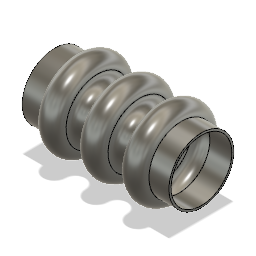
Table_13p3_Problem_6b (Autodesk Fusion 360 design; units mm, degrees)
Autodesk Fusion 360 part; units mm, degrees
sketch "Sketch1" plane through (0, 0, 0) normal (0, 0, 1) x (1, 0, 0)
  line L0 (0, 0) -> (0, 80) construction
  line L1 (0, 0) -> (10, 0) construction
  line L2 (10, 0) -> (80, 0) construction
  line L3 (140, 60) -> (100, 60) construction
  arc A0 (100, 60) -> (60, 60) centre (80, 60) ccw construction
  arc A1 (20, 60) -> (60, 60) centre (40, 60) ccw construction
  arc A2 (20, 60) -> (0, 80) centre (0, 60) ccw construction
  line L4 (140, 60) -> (0, 60) construction
  line L5 (140, 62) -> (101.9089, 62)
  arc A3 (101.9089, 62) -> (58, 60) centre (80, 60) ccw
  arc A4 (22, 60) -> (58, 60) centre (40, 60) ccw
  arc A5 (22, 60) -> (0, 82) centre (0, 60) ccw
  line L6 (140, 58) -> (97.8885, 58)
  arc A6 (97.8885, 58) -> (62, 60) centre (80, 60) ccw
  arc A7 (18, 60) -> (62, 60) centre (40, 60) ccw
  arc A8 (18, 60) -> (0, 78) centre (0, 60) ccw
  line L7 (140, 62) -> (140, 58)
  line L8 (-140, 58) -> (-97.8885, 58)
  line L9 (-140, 62) -> (-140, 58)
  line L10 (-140, 62) -> (-101.9089, 62)
  arc A9 (-58, 60) -> (-101.9089, 62) centre (-80, 60) ccw
  arc A10 (-62, 60) -> (-97.8885, 58) centre (-80, 60) ccw
  arc A11 (-62, 60) -> (-18, 60) centre (-40, 60) ccw
  arc A12 (-58, 60) -> (-22, 60) centre (-40, 60) ccw
  arc A13 (0, 82) -> (-22, 60) centre (0, 60) ccw
  arc A14 (0, 78) -> (-18, 60) centre (0, 60) ccw
  dimension "Shell_Thickness_1" = 2
  dimension "Shell_Thickness_2" = -2
  dimension "Toroid_Minor_Radius" = 20
  dimension "Toroid_Major_Radius" = 60
  dimension "Extension_Length" = 40
  constraint coincident L0.start L1.start
  constraint vertical L0
  constraint perpendicular L0 L1
  constraint perpendicular L0 L2
  constraint horizontal L3
  constraint tangent A0 A1
  constraint tangent A1 A2
  constraint equal A1 A2
  constraint equal A0 A1
  constraint coincident L0.end A2.end
  constraint coincident A2.centre L4.end
  constraint horizontal L4
  constraint coincident A1.centre L4
  constraint coincident A0.centre L4
  constraint coincident L0 A2.centre
  constraint perpendicular L6 L7
  constraint midpoint L3.start L7
  constraint symmetric L0 L5.start L9.start
  constraint symmetric L0 L5.end L10.end
  constraint symmetric L0 A3.end A9.start
  constraint symmetric L0 A3 A9
  constraint symmetric L0 A4.start A12.end
  constraint symmetric L0 A4 A12
  constraint symmetric L0 A5.end A13.start
  constraint symmetric L0 A5 A13
  constraint symmetric L0 L6.start L8.start
  constraint symmetric L0 L6.end L8.end
  constraint symmetric L0 A6.end A10.start
  constraint symmetric L0 A6 A10
  constraint symmetric L0 A7.start A11.end
  constraint symmetric L0 A7 A11
  constraint symmetric L0 A8.end A14.start
  constraint symmetric L0 A8 A14
  measures "Toroid_Minor_Radius" radius of A0
  measures "Toroid_Major_Radius" distance of L0.start A2.centre
  measures "Extension_Length" distance of L3.start L3.end
revolve "Revolve1" add sketch "Sketch1" angle 360 about axis through (10, 0, 0) along (1, 0, 0)
